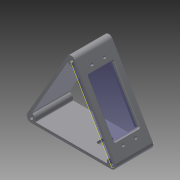
# Autodesk Inventor part: ServoHousing
Saved by Autodesk Inventor 2015 (Build 190159000, 159)
## iProperties
Created: 2014-11-03
Part Number: ServoHousing
Material: Generic
Document SubType Name: Modeling
Designer: rawrdong
Density: 1 g/cm^3
Appearance: Default
Author: rawrdong
Autodesk Inventor part; units mm, degrees
ref_plane "YZ Plane" through (0, 0, 0) normal (1, 0, 0) x (0, 1, 0)
ref_plane "XZ Plane" through (0, 0, 0) normal (0, 1, 0) x (-1, 0, 0)
ref_plane "XY Plane" through (0, 0, 0) normal (0, 0, 1) x (1, 0, 0)
sketch "Sketch2" plane through (0, 0, 0) normal (0, 1, 0) x (-1, 0, 0)
  circle A0 centre (0, 36.950417) radius 1.4
  circle A1 centre (0, 36.950417) radius 3.5
  circle A2 centre (-32, -18.475209) radius 1.4
  circle A3 centre (-32, -18.475209) radius 3.5
  circle A4 centre (32, -18.475209) radius 1.4
  circle A5 centre (32, -18.475209) radius 3.5
  line L0 (-35.031089, -16.725209) -> (-3.031089, 38.700417)
  line L1 (-2.717119, 34.744229) -> (-31.447945, -15.019021)
  line L2 (-32, -21.975209) -> (32, -21.975209)
  line L3 (35.031089, -16.725209) -> (3.031089, 38.700417)
  line L4 (-28.730826, -19.725209) -> (28.730826, -19.725209)
  line L5 (31.447945, -15.019021) -> (2.717119, 34.744229)
  line L6 (0, -21.975209) -> (0, -19.725209) construction
  line L7 (19.031089, 10.987604) -> (17.082532, 9.862604) construction
  line L8 (-17.082532, 9.862604) -> (-19.031089, 10.987604) construction
  line L9 (-5.434238, 30.038041) -> (-28.730826, -10.312833) construction
  line L10 (-28.730826, -10.312833) -> (-16.744911, -17.232904) construction
  line L11 (-16.744911, -17.232904) -> (6.551677, 23.11797) construction
  line L12 (6.551677, 23.11797) -> (-5.434238, 30.038041) construction
  point P0 (0, 0)
  point P1 (0, 0)
  dimension "d21" = 360
  dimension "d23" = 64
  dimension "d24" = 2.8
  dimension "d25" = 7
  dimension "d30" = 2.25
  dimension "d106" = 13.84014
  constraints: 26 end point, 12 point on circle, 6 centre point, 6 midpoint, 6 tangent, 5 parallel, 4 coincident, 2 equal length, 2 point on line, 1 horizontal, 1 perpendicular, 1 vertical alignment, 13 other
  measures "d23" distance of A4.centre A2.centre
  measures "d24" diameter of A2
  measures "d25" diameter of A3
  measures "d30" distance between parallel lines of L0 L1
  measures "d106" distance of L9.end L10.end
extrude "Extrusion3" add sketch "Sketch2" along normal blind 30 contours A1 | A1 L3 A5 L5 | A1 L1 A3 L0 | A5 | A3 | A5 L2 A3 L4
sketch "Servo1" plane through (35.031089, 0, -16.725209) normal (0.8660254, 0, 0.5) x (0.5, 0, -0.8660254)
  line L0 (-64, 30) -> (0, 30)
  line L1 (-53, 25.1) -> (-11, 25.1)
  line L2 (-11, 25.1) -> (-11, 4.9)
  line L3 (-11, 4.9) -> (-53, 4.9)
  line L4 (-53, 4.9) -> (-53, 25.1)
  circle A0 centre (-7, 20) radius 1.075
  circle A1 centre (-7, 10) radius 1.075
  line L5 (-32, 30) -> (-32, -15.528403)
  line L6 (-11, 15) -> (-53, 15) construction
  circle A2 centre (-57, 20) radius 1.075
  circle A3 centre (-57, 10) radius 1.075
  line L7 (0, 0) -> (0, 30)
  point P0 (-32, 0)
  point P1 (-32, 4.9)
  point P2 (0, 15)
  dimension "d43" = 2.15
  dimension "d44" = 20.2
  dimension "d45" = 42
  dimension "d47" = 50
  dimension "d96" = 10
  constraints: 12 end point, 5 midpoint, 4 centre point, 3 parallel, 3 symmetric about line, 1 equal radius, 1 horizontal, 1 horizontal alignment, 1 perpendicular, 1 point on line, 2 other
  measures "d43" diameter of A0
  measures "d44" distance of L3.end L1.start
  measures "d45" distance of L2.end L3.end
  measures "d47" diameter of A0.centre L5
  measures "d96" distance of A0.centre A1.centre
extrude "Extrusion4" cut sketch "Servo1" against normal blind 25 contours L1 L5 L3 L4 | L1 L2 L3 L5
extrude "Extrusion5" cut sketch "Servo1" against normal up to next contours A0 | A1 | A2 | A3
fillet "Fillet4" radius 0.8 4 edges at (7.5568, 25.1, 28.6116) (7.5568, 4.9, 28.6116) (28.5568, 4.9, -7.7614) (28.5568, 25.1, -7.7614)
ref_plane "Work Plane1" through (2.717119, 0, 34.744229) normal (-0.8660254, 0, -0.5) x (-0.5, 0, 0.8660254)
sketch "Sketch7" plane through (2.717119, 0, 34.744229) normal (-0.8660254, 0, -0.5) x (-0.5, 0, 0.8660254)
  line L0 (-7.730826, 5.7) -> (-7.730826, 24.3)
  line L1 (-8.530826, 25.1) -> (-48.930826, 25.1)
  arc A0 (-7.730826, 24.3) -> (-8.530826, 25.1) centre (-8.530826, 24.3) ccw
  arc A1 (-8.530826, 4.9) -> (-7.730826, 5.7) centre (-8.530826, 5.7) ccw
  line L2 (-48.930826, 4.9) -> (-8.530826, 4.9)
  arc A2 (-49.730826, 5.7) -> (-48.930826, 4.9) centre (-48.930826, 5.7) ccw
  line L3 (-49.730826, 24.3) -> (-49.730826, 5.7)
  arc A3 (-48.930826, 25.1) -> (-49.730826, 24.3) centre (-48.930826, 24.3) ccw
  line L4 (-48.930826, 27.6) -> (-8.530826, 27.6)
  arc A4 (-5.230826, 24.3) -> (-8.530826, 27.6) centre (-8.530826, 24.3) ccw
  line L5 (-5.230826, 24.3) -> (-5.230826, 5.7)
  arc A5 (-8.530826, 2.4) -> (-5.230826, 5.7) centre (-8.530826, 5.7) ccw
  line L6 (-8.530826, 2.4) -> (-48.930826, 2.4)
  arc A6 (-52.230826, 5.7) -> (-48.930826, 2.4) centre (-48.930826, 5.7) ccw
  line L7 (-52.230826, 5.7) -> (-52.230826, 24.3)
  arc A7 (-48.930826, 27.6) -> (-52.230826, 24.3) centre (-48.930826, 24.3) ccw
  line L8 (-52.230826, 24.3) -> (-61.176721, 24.3)
  line L9 (-61.176721, 24.3) -> (-61.176721, 5.7)
  line L10 (-52.230826, 5.7) -> (-61.176721, 5.7)
  line L11 (-28.730826, 4.9) -> (-28.730826, 25.1) construction
  line L12 (-5.230826, 24.3) -> (3.715069, 24.3)
  line L13 (3.715069, 24.3) -> (3.715069, 5.7)
  line L14 (-5.230826, 5.7) -> (3.715069, 5.7)
  circle A8 centre (-53.730826, 20) radius 1.075
  circle A9 centre (-53.730826, 10) radius 1.075
  circle A10 centre (-3.730826, 10) radius 1.075
  circle A11 centre (-3.730826, 20) radius 1.075
  dimension "d82" = 2.5
  constraints: 22 end point, 8 point on circle, 4 centre point, 3 perpendicular, 2 horizontal, 2 midpoint, 1 vertical, 8 other
  measures "d82" distance between parallel lines of L4 L1
extrude "Extrusion8" add sketch "Sketch7" along normal blind 2
fillet "Fillet6" radius 2 4 edges at (27.9665, 24.3, -10.989) (4.4665, 24.3, 29.7142) (4.4665, 5.7, 29.7142) (27.9665, 5.7, -10.989)
chamfer "Chamfer2" distance 2 angle 45 14 edges at (17.0825, 27.6, 9.8626) (6.0619, 27.0386, 28.9509) (5.0864, 24.6403, 30.6405) (3.6228, 24.3, 33.1756) (28.1032, 27.0386, -9.2257) (29.0786, 24.6403, -10.9153) (30.5423, 24.3, -13.4504) (17.0825, 2.4, 9.8626) (28.1032, 2.9614, -9.2257) (29.0786, 5.3597, -10.9153) (30.5423, 5.7, -13.4504) (6.0619, 2.9614, 28.9509) (5.0864, 5.3597, 30.6405) (3.6228, 5.7, 33.1756)
fillet "Fillet7" radius 0.5 8 edges at (2.7171, 1.8501, 34.7442) (-2.7171, 15, 34.7442) (2.7171, 28.1499, 34.7442) (-31.4479, 15, -15.019) (-28.7308, 15, -19.7252) (28.7308, 15, -19.7252) (31.4479, 1.85, -15.019) (31.4479, 28.1499, -15.019)
chamfer "Chamfer3" distance 0.5 angle 45 8 edges at (19.0311, 4.9, 10.9876) (8.6482, 5.1343, 28.9712) (8.5311, 15, 29.1741) (8.6482, 24.8657, 28.9712) (19.0311, 25.1, 10.9876) (29.4139, 24.8657, -6.996) (29.5311, 15, -7.1989) (29.4139, 5.1343, -6.996)
sketch "Sketch9" plane through (32, 0, -21.975209) normal (0, 0, -1) x (-1, 0, 0)
  line L0 (0, 0) -> (0, 30)
  line L1 (17.5, 20) -> (22.5, 20)
  line L2 (22.5, 20) -> (22.5, 10)
  line L3 (22.5, 10) -> (17.5, 10)
  line L4 (17.5, 10) -> (17.5, 20)
  line L5 (0, 15) -> (22.5, 15) construction
  point P0 (-33.5, 0)
  dimension "d97" = 5
  dimension "d98" = 10
  dimension "d104" = 22.5
  constraints: 12 end point, 2 horizontal, 2 midpoint, 2 parallel, 1 perpendicular
  measures "d97" distance of L1.start L1.end
  measures "d98" distance of L3.end L1.start
  measures "d104" distance of L5.start L5.end
extrude "Extrusion9" cut sketch "Sketch9" against normal up to surface surface through (-2.717119, 0, 34.744229) normal (0.8660254, 0, -0.5)
fillet "Fillet8" radius 1.5 4 edges at (9.5, 20, -20.8502) (14.5, 20, -20.8502) (14.5, 10, -20.8502) (9.5, 10, -20.8502)
body "Solid2"
body "Solid3"
